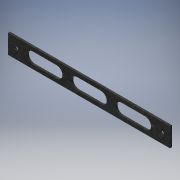
# Autodesk Inventor part: transverseClipStiffener
Saved by Autodesk Inventor 2016 (Build 200138000, 138)
## iProperties
Created: 2015-11-15
Part Number: transverseClipStiffener
Material: Steel
Document SubType Name: Modeling
Designer: Artur
Density: 7.85 g/cm^3
Appearance: Plate
Mass: 38.3733 g
Surface Area: 63.1791 cm^2
Volume: 4.88832 cm^3
Author: Artur
Autodesk Inventor part; units mm, degrees
ref_plane "YZ Plane" through (0, 0, 0) normal (1, 0, 0) x (0, 1, 0)
ref_plane "XZ Plane" through (0, 0, 0) normal (0, 1, 0) x (-1, 0, 0)
ref_plane "XY Plane" through (0, 0, 0) normal (0, 0, 1) x (1, 0, 0)
sketch "Sketch1" plane through (0, 0, 0) normal (0, 1, 0) x (-1, 0, 0)
  line L0 (0, 0) -> (169, 0)
  line L1 (169, 0) -> (169, -20)
  line L2 (169, -20) -> (0, -20)
  line L3 (0, -20) -> (0, 0)
  dimension "d0" = 169
  dimension "d1" = 20
  constraints: 8 end point, 2 parallel, 1 horizontal, 1 perpendicular
  measures "d0" distance of L1.end L2.end
  measures "d1" distance of L0.end L1.end
extrude "base" add sketch "Sketch1" along normal blind 2
sketch "Sketch2" plane through (0, 0, 0) normal (0, -1, 0) x (1, 0, 0)
  circle A0 centre (-160.5, -10) radius 2
  circle A1 centre (-8.5, -10) radius 2
  line L0 (-169, -20) -> (-169, 0) construction
  line L1 (-169, -10) -> (0, -10) construction
  line L2 (0, 0) -> (0, -20) construction
  dimension "d4" = 152
  dimension "d5" = 4
  dimension "d6" = 4
  dimension "d7" = 8.5
  dimension "d8" = 169
  constraints: 2 centre point, 2 end point, 2 midpoint, 2 point on line
  measures "d4" distance of A1.centre A0.centre
  measures "d5" diameter of A1
  measures "d6" diameter of A0
  measures "d7" distance from line of L0 A0.centre
  measures "d8" distance between parallel lines of L2 L0
extrude "holes" cut sketch "Sketch2" against normal blind 2
sketch "Sketch3" plane through (0, 0, 0) normal (0, -1, 0) x (1, 0, 0)
  line L0 (0, 0) -> (0, -20) construction
  line L1 (0, -10) -> (-169, -10) construction
  line L2 (-169, -20) -> (-169, 0) construction
  circle A0 centre (-160.5, -10) radius 2 construction
  line L3 (-160.5, -10) -> (-160.5, 5.7595) construction
  circle A1 centre (-8.5, -10) radius 2 construction
  line L4 (-8.5, -10) -> (-8.5, 9.069) construction
  arc A2 (-143.25, -4) -> (-143.25, -16) centre (-143.25, -10) ccw
  line L5 (-143.25, -10) -> (-143.25, -16) construction
  line L6 (-143.25, -10) -> (-143.25, -4) construction
  line L7 (-143.25, -4) -> (-118.25, -4)
  line L8 (-143.25, -16) -> (-118.25, -16)
  arc A3 (-118.25, -16) -> (-118.25, -4) centre (-118.25, -10) ccw
  line L9 (-118.25, -10) -> (-118.25, -16) construction
  line L10 (-118.25, -10) -> (-118.25, -4) construction
  line L11 (-97, -4) -> (-72, -4)
  arc A4 (-97, -4) -> (-97, -16) centre (-97, -10) ccw
  line L12 (-97, -16) -> (-72, -16)
  arc A5 (-72, -16) -> (-72, -4) centre (-72, -10) ccw
  line L13 (-50.75, -4) -> (-25.75, -4)
  arc A6 (-50.75, -4) -> (-50.75, -16) centre (-50.75, -10) ccw
  line L14 (-50.75, -16) -> (-25.75, -16)
  arc A7 (-25.75, -16) -> (-25.75, -4) centre (-25.75, -10) ccw
  point P0 (-158.5, -10)
  point P1 (-10.5, -10)
  point P2 (-149.25, -10)
  dimension "d11" = 180
  dimension "d12" = 6
  dimension "d13" = 180
  dimension "d14" = 25
  dimension "d18" = 46.25
  dimension "d23" = 148
  dimension "d25" = 9.25
  constraints: 26 end point, 13 point on circle, 6 centre point, 3 horizontal, 3 point on line, 2 horizontal alignment, 2 midpoint, 2 vertical, 1 collinear, 1 parallel, 1 perpendicular, 21 other
  measures "d11" angle of L5 L6
  measures "d12" distance of L5.start L6.end
  measures "d13" angle of L9 L10
  measures "d14" distance of L6.end L7.end
  measures "d18" distance of L6.end L11.start
  measures "d23" distance of point (-10.5, -10) point (-158.5, -10)
  measures "d25" distance of point (-149.25, -10) point (-158.5, -10)
extrude "Extrusion3" cut sketch "Sketch3" against normal blind 10
equation "\"d6\" = d5"
equation "\"d7\" = -0.5 * d4 + 0.5 * d8"
equation "\"d18\" = 2 * d12 + d25 + d14"
equation "\"d25\" = -1.5 * d12 - 0.75 * d14 + 0.25 * d23"
equation "\"d24\" = -1.5 * d12 - 0.75 * d14 + 0.25 * d23"
body "Solid1"
